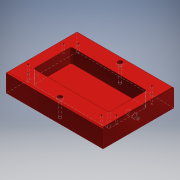
# Autodesk Inventor part: UNLHEP-14-01-P-004_ChuckForGantry
Saved by Autodesk Inventor 2019.4 (Build 234330000, 330)
## iProperties
Created: 2014-01-09
Part Number: UNLHEP-14-01-P-004_ChuckForGantry
Material: Aluminum, Anodized Red
Document SubType Name: Modeling
Designer: Frank Meier
Density: 2.7 g/cm^3
Project: UNL Pixel Phase I
Mass: 2699.72 g
Surface Area: 1115.91 cm^2
Volume: 999.896 cm^3
Appearance: Anodized - Red
Author: Frank Meier
Revision Number: 00
Autodesk Inventor part; units mm, degrees
ref_plane "YZ Plane" through (0, 0, 0) normal (1, 0, 0) x (0, 1, 0)
ref_plane "XZ Plane" through (0, 0, 0) normal (0, 1, 0) x (-1, 0, 0)
ref_plane "XY Plane" through (0, 0, 0) normal (0, 0, 1) x (1, 0, 0)
sketch "Skizze1" plane through (0, 0, 0) normal (0, 0, 1) x (1, 0, 0)
  line L0 (-123, -90) -> (123, -90)
  line L1 (123, -90) -> (123, 90)
  line L2 (123, 90) -> (-123, 90)
  line L3 (-123, 90) -> (-123, -90)
  line L4 (-123, -90) -> (123, 90) construction
  line L5 (123, -90) -> (-123, 90) construction
  point P0 (0, 0)
  dimension "d0" = 246
  dimension "d2" = 180
  constraints: 12 end point, 2 midpoint, 2 parallel, 1 horizontal, 1 perpendicular
  measures "d0" distance of L1.end L2.end
  measures "d2" distance of L0.end L1.end
extrude "Extrusion1" add sketch "Skizze1" along normal blind 46
sketch "Skizze2" plane through (0, 0, 46) normal (0, 0, 1) x (1, 0, 0)
  line L0 (-96, -48) -> (96, -48)
  line L1 (96, -48) -> (96, 48)
  line L2 (96, 48) -> (-96, 48)
  line L3 (-96, 48) -> (-96, -48)
  line L4 (-96, -48) -> (96, 48) construction
  line L5 (96, -48) -> (-96, 48) construction
  line L6 (-123, -90) -> (123, -90) projected
  line L7 (123, -90) -> (123, 90) projected
  line L8 (123, 90) -> (-123, 90) projected
  line L9 (-123, 90) -> (-123, -90) projected
  circle A0 centre (-115, 60) radius 2
  circle A1 centre (-93, 82) radius 2
  circle A2 centre (93, 82) radius 2
  circle A3 centre (115, 60) radius 2
  circle A4 centre (115, -60) radius 2
  circle A5 centre (93, -82) radius 2
  circle A6 centre (-93, -82) radius 2
  circle A7 centre (-115, -60) radius 2
  point P0 (0, 0)
  dimension "d5" = 192
  dimension "d7" = 96
  dimension "d14" = 8
  dimension "d15" = 30
  dimension "d16" = 30
  dimension "d17" = 8
  dimension "d18" = 8
  dimension "d19" = 30
  dimension "d20" = 8
  dimension "d21" = 30
  dimension "d22" = 30
  dimension "d23" = 8
  dimension "d24" = 8
  dimension "d25" = 30
  dimension "d26" = 8
  dimension "d27" = 30
  dimension "d28" = 30
  dimension "d29" = 8
  dimension "d30" = 4
  dimension "d31" = 4
  dimension "d32" = 4
  dimension "d33" = 4
  dimension "d34" = 4
  dimension "d35" = 4
  dimension "d36" = 4
  dimension "d37" = 4
  constraints: 12 end point, 8 centre point, 8 coincident, 2 midpoint, 2 parallel, 1 horizontal, 1 perpendicular
  measures "d5" distance of L1.end L2.end
  measures "d7" distance of L0.end L1.end
  measures "d14" distance from line of L9 point (-115, 60)
  measures "d15" distance from line of L8 point (-115, 60)
  measures "d16" distance from line of L9 point (-93, 82)
  measures "d17" distance from line of L8 point (-93, 82)
  measures "d18" distance from line of L8 point (93, 82)
  measures "d19" distance from line of L7 point (93, 82)
  measures "d20" distance from line of L7 point (115, 60)
  measures "d21" distance from line of L8 point (115, 60)
  measures "d22" distance from line of L6 point (115, -60)
  measures "d23" distance from line of L7 point (115, -60)
  measures "d24" distance from line of L6 point (93, -82)
  measures "d25" distance from line of L7 point (93, -82)
  measures "d26" distance from line of L6 point (-93, -82)
  measures "d27" distance from line of L9 point (-93, -82)
  measures "d28" distance from line of L6 point (-115, -60)
  measures "d29" distance from line of L9 point (-115, -60)
  measures "d30" diameter of A0
  measures "d31" diameter of A1
  measures "d32" diameter of A2
  measures "d33" diameter of A3
  measures "d34" diameter of A4
  measures "d35" diameter of A5
  measures "d36" diameter of A6
  measures "d37" diameter of A7
extrude "Extrusion2" cut sketch "Skizze2" against normal blind 36 contours L3 L2 L1 L0
fillet "Rundung1" radius 4 4 edges at (-96, 48, 28) (96, 48, 28) (96, -48, 28) (-96, -48, 28)
chamfer "Fase1" distance 2 angle 45 4 edges at (0, -90, 46) (-123, 0, 46) (0, 90, 46) (123, 0, 46)
sketch "Skizze4" plane through (0, 0, 46) normal (0, 0, 1) x (1, 0, 0)
  line L0 (123, 90) -> (-123, 90) projected
  line L1 (123, -90) -> (123, 90) projected
  line L2 (-123, 90) -> (-123, -90) projected
  line L3 (-123, -90) -> (123, -90) projected
  point P0 (-112, 45)
  point P1 (-112, -45)
  point P2 (-93, -64)
  point P3 (-93, 64)
  point P4 (93, 64)
  point P5 (112, 45)
  point P6 (112, -45)
  point P7 (93, -64)
  dimension "d153" = 45
  dimension "d154" = 45
  dimension "d155" = 11
  dimension "d156" = 26
  dimension "d157" = 30
  dimension "d158" = 11
  dimension "d159" = 26
  dimension "d160" = 30
  dimension "d161" = 30
  dimension "d162" = 26
  dimension "d163" = 11
  dimension "d164" = 45
  dimension "d165" = 11
  dimension "d166" = 45
  dimension "d167" = 26
  dimension "d168" = 30
  measures "d153" distance from line of L0 point (-112, 45)
  measures "d154" distance from line of L3 point (-112, -45)
  measures "d155" distance from line of L2 point (-112, -45)
  measures "d156" distance from line of L3 point (-93, -64)
  measures "d157" distance from line of L2 point (-93, -64)
  measures "d158" distance from line of L2 point (-112, 45)
  measures "d159" distance from line of L0 point (-93, 64)
  measures "d160" distance from line of L2 point (-93, 64)
  measures "d161" distance from line of L1 point (93, 64)
  measures "d162" distance from line of L0 point (93, 64)
  measures "d163" distance from line of L1 point (112, 45)
  measures "d164" distance from line of L0 point (112, 45)
  measures "d165" distance from line of L1 point (112, -45)
  measures "d166" distance from line of L3 point (112, -45)
  measures "d167" distance from line of L3 point (93, -64)
  measures "d168" distance from line of L1 point (93, -64)
sketch "Sketch10" plane through (123, -90, 0) normal (1, 0, 0) x (0, 0, -1)
  line L0 (-46, 178) -> (-46, 2) projected
  line L1 (0, 0) -> (-44, 0) projected
  point P0 (-23, 90)
  dimension "d92" = 23
  dimension "d93" = 90
  measures "d92" distance from line of L0 point (-23, 90)
  measures "d93" distance from line of L1 point (-23, 90)
hole "Bohrung3" at (123, 0, 23) direction (-1, 0, 0) diameter 10.719 depth 27 tip angle 118 taper from width 11.358 to width 10.732 over 10.02 thread size "1/4" designation "1/4 - 18 NPT" standard "NPT"
sketch "Skizze9" plane through (0, 0, 46) normal (0, 0, 1) x (1, 0, 0)
  line L0 (123, 90) -> (-123, 90) projected
  point P0 (0, 0)
  point P1 (0, 76.2)
  point P2 (0, -76.2)
  dimension "d143" = 152.4
  dimension "d145" = 13.8
  measures "d143" distance of point (0, -76.2) point (0, 76.2)
  measures "d145" distance from line of L0 point (0, 76.2)
hole "Bohrung6" at (0, 76.2, 46) at (0, -76.2, 46) direction (0, 0, -1) diameter 6.756 depth 50 tip angle 118 counterbore diameter 11.113 counterbore depth 6.35 clearance for "Innensechskantkopfschraube" size "1/4" standard "ANSI UST"
hole "Bohrung7" at (-112, 45, 46) at (-112, -45, 46) at (-93, -64, 46) at (-93, 64, 46) at (93, 64, 46) at (112, 45, 46) at (112, -45, 46) at (93, -64, 46) direction (0, 0, -1) diameter 3.242 depth 20 tip angle 118 thread size "M4x0.7" class "6H" standard "ISO Metric profile"
